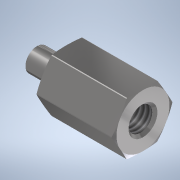
# Autodesk Inventor part: MSU-308-03
Saved by Autodesk Inventor 2020 (Build 240168000, 168)
## iProperties
Created: 2016-05-27
Part Number: MSU-308-03
Document SubType Name: Modeling
Manufacturer: MISUMI
Mass: 1.52544 g
Surface Area: 2.75206 cm^2
Volume: 0.19068 cm^3
Density: 8 g/cm^3
Material: ステンレス鋼 AISI 302
Appearance: 半つや出し
Title: MSU-308-03
Autodesk Inventor part; units mm, degrees
ref_plane "YZ Plane" through (0, 0, 0) normal (1, 0, 0) x (0, 1, 0)
ref_plane "XZ Plane" through (0, 0, 0) normal (0, 1, 0) x (-1, 0, 0)
ref_plane "XY Plane" through (0, 0, 0) normal (0, 0, 1) x (1, 0, 0)
sketch "Sketch_1" plane through (0, 0, 0) normal (0, 0, 1) x (1, 0, 0)
  line L0 (8, 0) -> (0, 0)
  line L1 (0, 0) -> (0, 2.75)
  line L2 (0, 2.75) -> (0.1072, 3.15)
  line L3 (0.1072, 3.15) -> (7.8928, 3.15)
  line L4 (7.8928, 3.15) -> (8, 2.75)
  line L5 (8, 2.75) -> (8, 0)
  line L6 (8, 0) -> (0, 0)
  constraints: 14 end point
revolve "Revolution1" add sketch "Sketch_1" angle 360 about axis through (8, 0, 0) along (1, 0, 0)
sketch "Sketch_5" plane through (0, 0, 0) normal (0, 0, 1) x (1, 0, 0)
  line L0 (0, 0) -> (-6, 0)
  line L1 (-6, 0) -> (-6, 1.1935)
  line L2 (-6, 1.1935) -> (-5.6935, 1.5)
  line L3 (-5.6935, 1.5) -> (-0.6, 1.5)
  line L4 (-0.6, 1.5) -> (-0.6, 1.2295)
  line L5 (-0.6, 1.2295) -> (0, 1.2295)
  line L6 (0, 1.2295) -> (0, 0)
  line L7 (0, 0) -> (-6, 0)
  constraints: 16 end point
revolve "Revolution2" add sketch "Sketch_5" angle 360 about axis through (0, 0, 0) along (1, 0, 0)
thread "Thread1" size "M3x0.5" class "6g" standard "ISO Metric profile" full length
sketch "Sketch_6" plane through (0, 0, 0) normal (1, 0, 0) x (0, 1, 0)
  circle A0 centre (0, 0) radius 6.3
  line L0 (1.5877, 2.75) -> (-1.5877, 2.75)
  line L1 (-1.5877, 2.75) -> (-3.1754, 0)
  line L2 (-3.1754, 0) -> (-1.5877, -2.75)
  line L3 (-1.5877, -2.75) -> (1.5877, -2.75)
  line L4 (1.5877, -2.75) -> (3.1754, 0)
  line L5 (3.1754, 0) -> (1.5877, 2.75)
  constraints: 12 end point, 1 centre point
extrude "Extrusion1" cut sketch "Sketch_6" along normal blind 8
sketch "Sketch4" plane through (8, 0, 0) normal (1, 0, 0) x (0, 0, -1)
  point P0 (0, 0)
hole "Hole1" at (8, 0, 0) direction (-1, 0, 0) diameter 2.459 depth 6.4901 tip angle 120 countersink diameter 3 countersink angle 90 thread size "M3x0.5" class "6H" standard "ISO Metric profile"
sketch "スケッチ5" plane through (-6, 0, 0) normal (-1, 0, 0) x (0, 0, 1)
  circle A0 centre (0, 0) radius 1.1935 projected
  circle A1 centre (0, 0) radius 1.2
  circle A2 centre (0, 0) radius 2.2848
  dimension "d13" = 2.4
  constraints: 2 centre point, 2 coincident
  measures "d13" diameter of A1
extrude "押し出し2" cut sketch "スケッチ5" against normal blind 6 contours A2
sketch "スケッチ6" plane through (-6, 0, 0) normal (-1, 0, 0) x (0, 0, 1)
  circle A0 centre (0, 0) radius 1.1935 projected
  circle A1 centre (0, 0) radius 1.9337
  constraints: 1 centre point, 1 coincident
extrude "押し出し3" cut sketch "スケッチ6" against normal blind 3 contours A0 | A1
body "Solid1"
